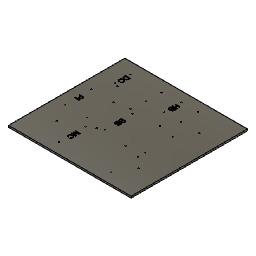
Bigger Board Tester v1 (Autodesk Fusion 360 design; units mm, degrees)
Autodesk Fusion 360 part; units mm, degrees
sketch "Sketch1" plane through (0, 0, 0) normal (0, 0, 1) x (1, 0, 0)
  circle A0 centre (-13.6792, 145.0658) radius 1.5
  circle A1 centre (165.3208, 145.0658) radius 1.5
  circle A2 centre (-13.6792, 12.1658) radius 1.5
  circle A3 centre (165.3208, 12.1658) radius 1.5
  circle A4 centre (43.3208, 42.5182) radius 1.5
  circle A5 centre (108.3208, 41.4658) radius 1.5
  circle A6 centre (43.3208, 116.7382) radius 1.5
  circle A7 centre (108.3208, 115.7658) radius 1.5
  line L0 (-58.5792, 206.1658) -> (210.2208, 206.1658)
  line L1 (210.2208, 206.1658) -> (210.2208, -48.9342)
  line L2 (210.2208, -48.9342) -> (-58.5792, -48.9342)
  line L3 (-58.5792, -48.9342) -> (-58.5792, 206.1658)
  dimension "d1" = 3
  dimension "d2" = 3
  dimension "d3" = 3
  dimension "d4" = 3
  dimension "d15" = 3
  dimension "d16" = 3
  dimension "d17" = 3
  dimension "d21" = 74.3
  dimension "d36" = 65
  dimension "d38" = 65
  dimension "d97" = 132.9
  dimension "d98" = 132.9
  dimension "d99" = 179
  dimension "d100" = 179
  dimension "d101" = 57
  dimension "d102" = 28.3275
  dimension "d106" = 61.1
  dimension "d107" = 61.1
  dimension "d108" = 44.9
  dimension "d109" = 44.9
  constraint horizontal L0
  constraint vertical L1
  constraint horizontal L2
  constraint vertical L3
  measures "d1" diameter of A0
  measures "d2" diameter of A1
  measures "d3" diameter of A2
  measures "d4" diameter of A3
  measures "d15" diameter of A5
  measures "d16" diameter of A6
  measures "d17" diameter of A7
  measures "d21" vertical distance of A5.centre A7.centre
  measures "d36" horizontal distance of A4.centre A5.centre
  measures "d38" horizontal distance of A6.centre A7.centre
  measures "d97" distance of A0.centre A2.centre
  measures "d98" distance of A1.centre A3.centre
  measures "d99" distance of A0.centre A1.centre
  measures "d100" distance of A2.centre A3.centre
  measures "d101" horizontal distance of A0.centre A6.centre
  measures "d102" vertical distance of A0.centre A6.centre
  measures "d106" distance of A2.centre L2
  measures "d107" distance of A0.centre L0
  measures "d108" distance of A0.centre L3
  measures "d109" distance of A1.centre L1
extrude "Extrude1" add sketch "Sketch1" along normal blind 3.5
sketch "Sketch2" plane through (0, 0, 3.5) normal (0, 0, 1) x (-1, 0, 0)
  circle A0 centre (-43.3208, -116.7382) radius 1.5
  circle A1 centre (-165.3208, -12.1658) radius 1.5
  circle A2 centre (-108.3208, -41.4658) radius 1.5
  circle A3 centre (13.6792, -12.1658) radius 1.5
  circle A4 centre (13.6792, -145.0658) radius 1.5
  circle A5 centre (-43.3208, -42.5182) radius 1.5
  circle A6 centre (-108.3208, -115.7658) radius 1.5
  circle A7 centre (-165.3208, -145.0658) radius 1.5
  line L0 (58.5792, 48.9342) -> (-210.2208, 48.9342)
  line L1 (-210.2208, 48.9342) -> (-210.2208, -206.1658)
  line L2 (-210.2208, -206.1658) -> (58.5792, -206.1658)
  line L3 (58.5792, -206.1658) -> (58.5792, 48.9342)
  line L4 (38.7881, -112.7975) -> (-15.0119, -112.7975)
  line L5 (-15.0119, -112.7975) -> (-15.0119, -49.6975)
  line L6 (-15.0119, -49.6975) -> (38.7881, -49.6975)
  line L7 (38.7881, -49.6975) -> (38.7881, -112.7975)
  circle A8 centre (36.2881, -110.2975) radius 1.25
  circle A9 centre (36.2881, -52.1975) radius 1.25
  circle A10 centre (-12.5119, -52.1975) radius 1.25
  circle A11 centre (-12.5119, -110.2975) radius 1.25
  line L8 (-145.573, 28.0042) -> (-25.813, 28.0042)
  line L9 (-145.573, -35.8758) -> (-145.573, 28.0042)
  circle A12 centre (-143.073, 25.5042) radius 1.25
  line L10 (-25.813, 28.0042) -> (-25.813, -35.8758)
  circle A13 centre (-143.073, -33.3758) radius 1.25
  circle A14 centre (-28.313, 25.5042) radius 1.25
  line L11 (-25.813, -35.8758) -> (-145.573, -35.8758)
  circle A15 centre (-28.313, -33.3758) radius 1.25
  line L12 (-125.9916, -186.7322) -> (-125.9916, -144.2322)
  line L13 (-84.6916, -186.7322) -> (-125.9916, -186.7322)
  circle A16 centre (-123.4916, -184.2322) radius 1.25
  line L14 (-125.9916, -144.2322) -> (-84.6916, -144.2322)
  circle A17 centre (-87.1916, -184.2322) radius 1.25
  circle A18 centre (-123.4916, -146.7322) radius 1.25
  line L15 (-84.6916, -144.2322) -> (-84.6916, -186.7322)
  circle A19 centre (-87.1916, -146.7322) radius 1.25
  line L16 (-145.6799, -111.5696) -> (-145.6799, -46.5696)
  line L17 (-52.6799, -111.5696) -> (-145.6799, -111.5696)
  circle A20 centre (-143.1799, -109.0696) radius 1.25
  line L18 (-145.6799, -46.5696) -> (-52.6799, -46.5696)
  circle A21 centre (-55.1799, -109.0696) radius 1.25
  circle A22 centre (-143.1799, -49.0696) radius 1.25
  line L19 (-52.6799, -46.5696) -> (-52.6799, -111.5696)
  circle A23 centre (-55.1799, -49.0696) radius 1.25
  line L20 (-49.2456, -183.6533) -> (-49.2456, -145.1533)
  line L21 (24.2544, -183.6533) -> (-49.2456, -183.6533)
  circle A24 centre (-46.7456, -181.1533) radius 1.25
  line L22 (-49.2456, -145.1533) -> (24.2544, -145.1533)
  circle A25 centre (21.7544, -181.1533) radius 1.25
  circle A26 centre (-46.7456, -147.6533) radius 1.25
  line L23 (24.2544, -145.1533) -> (24.2544, -183.6533)
  circle A27 centre (21.7544, -147.6533) radius 1.25
  dimension "d110" = 2.5
  dimension "d111" = 2.5
  dimension "d113" = 2.5
  dimension "d117" = 2.5
  dimension "d118" = 2.5
  dimension "d119" = 2.5
  dimension "d120" = 2.5
  dimension "d121" = 2.5
  dimension "d124" = 2.5
  dimension "d125" = 2.5
  dimension "d126" = 2.5
  dimension "d127" = 58.1
  dimension "d128" = 48.8
  dimension "d129" = 48.8
  dimension "d130" = 2.5
  dimension "d131" = 2.5
  dimension "d132" = 2.5
  dimension "d133" = 2.5
  dimension "d134" = 2.5
  dimension "d135" = 2.5
  dimension "d136" = 2.5
  dimension "d137" = 2.5
  dimension "d138" = 2.5
  dimension "d139" = 2.5
  dimension "d140" = 2.5
  dimension "d141" = 114.76
  dimension "d142" = 58.88
  dimension "d143" = 58.88
  dimension "d144" = 2.5
  dimension "d145" = 2.5
  dimension "d146" = 2.5
  dimension "d147" = 2.5
  dimension "d148" = 2.5
  dimension "d149" = 2.5
  dimension "d150" = 2.5
  dimension "d151" = 2.5
  dimension "d152" = 2.5
  dimension "d153" = 2.5
  dimension "d154" = 2.5
  dimension "d155" = 37.5
  dimension "d156" = 36.3
  dimension "d157" = 36.3
  dimension "d158" = 2.5
  dimension "d159" = 2.5
  dimension "d160" = 2.5
  dimension "d161" = 2.5
  dimension "d162" = 2.5
  dimension "d163" = 2.5
  dimension "d164" = 2.5
  dimension "d165" = 2.5
  dimension "d166" = 2.5
  dimension "d167" = 2.5
  dimension "d168" = 2.5
  dimension "d169" = 60
  dimension "d170" = 88
  dimension "d171" = 88
  dimension "d172" = 2.5
  dimension "d173" = 2.5
  dimension "d174" = 2.5
  dimension "d175" = 2.5
  dimension "d176" = 2.5
  dimension "d177" = 2.5
  dimension "d178" = 2.5
  dimension "d179" = 2.5
  dimension "d180" = 2.5
  dimension "d181" = 2.5
  dimension "d182" = 2.5
  dimension "d183" = 33.5
  dimension "d184" = 68.5
  dimension "d185" = 68.5
  dimension "d186" = 10
  dimension "d187" = 10
  dimension "d188" = 10
  dimension "d189" = 10
  dimension "d190" = 10
  dimension "d198" = 2.5
  dimension "d199" = 114.76
  text T0 "PI" font "Arial" height 10 align centre spacing 1 along the path L7 letters at x, y, angle (26.1414, -87.8471, 90) (26.1414, -78.5292, 90)
  text T1 "DC" font "Arial" height 10 align centre spacing 1 along the path L23 letters at x, y, angle (11.6077, -174.492, 90) (11.6077, -164.4033, 90)
  text T2 "HB" font "Arial" height 10 align centre spacing 1 along the path L15 letters at x, y, angle (-97.3383, -175.1855, 90) (-97.3383, -165.0968, 90)
  text T3 "BB" font "Arial" height 10 align centre spacing 1 along the path L19 letters at x, y, angle (-65.3266, -88.3874, 90) (-65.3266, -79.0696, 90)
  text T4 "MC" font "Arial" height 10 align centre spacing 1 along the path L10 letters at x, y, angle (-38.4596, -14.7987, 90) (-38.4596, -3.1616, 90)
  constraint horizontal L4
  constraint vertical L5
  constraint horizontal L6
  constraint vertical L7
  constraint horizontal L13
  constraint vertical L12
  constraint horizontal L14
  constraint vertical L15
  constraint horizontal L17
  constraint vertical L16
  constraint horizontal L18
  constraint vertical L19
  constraint horizontal L21
  constraint vertical L20
  constraint horizontal L22
  constraint vertical L23
  measures "d110" diameter of A8
  measures "d111" diameter of A9
  measures "d113" diameter of A10
  measures "d117" distance of L4 A8.centre
  measures "d118" distance of L7 A8.centre
  measures "d119" diameter of A11
  measures "d120" distance of L4 A11.centre
  measures "d121" distance of L5 A11.centre
  measures "d124" distance of L7 A9.centre
  measures "d125" distance of L6 A9.centre
  measures "d126" distance of L6 A10.centre
  measures "d127" distance of A8.centre A9.centre
  measures "d128" distance of A8.centre A11.centre
  measures "d129" distance of A9.centre A10.centre
  measures "d130" diameter of A13
  measures "d131" diameter of A15
  measures "d132" diameter of A14
  measures "d133" distance of A13.centre L9
  measures "d134" distance of A13.centre L11
  measures "d135" diameter of A12
  measures "d136" distance of A12.centre L9
  measures "d137" distance of A12.centre L8
  measures "d138" distance of A15.centre L11
  measures "d139" distance of A15.centre L10
  measures "d140" distance of A14.centre L10
  measures "d141" distance of A13.centre A15.centre
  measures "d142" distance of A12.centre A13.centre
  measures "d143" distance of A14.centre A15.centre
  measures "d144" diameter of A17
  measures "d145" diameter of A19
  measures "d146" diameter of A18
  measures "d147" distance of A17.centre L13
  measures "d148" distance of A17.centre L15
  measures "d149" diameter of A16
  measures "d150" distance of A16.centre L13
  measures "d151" distance of A16.centre L12
  measures "d152" distance of A19.centre L15
  measures "d153" distance of A19.centre L14
  measures "d154" distance of A18.centre L14
  measures "d155" distance of A17.centre A19.centre
  measures "d156" distance of A16.centre A17.centre
  measures "d157" distance of A18.centre A19.centre
  measures "d158" diameter of A21
  measures "d159" diameter of A23
  measures "d160" diameter of A22
  measures "d161" distance of A21.centre L17
  measures "d162" distance of A21.centre L19
  measures "d163" diameter of A20
  measures "d164" distance of A20.centre L17
  measures "d165" distance of A20.centre L16
  measures "d166" distance of A23.centre L19
  measures "d167" distance of A23.centre L18
  measures "d168" distance of A22.centre L18
  measures "d169" distance of A21.centre A23.centre
  measures "d170" distance of A20.centre A21.centre
  measures "d171" distance of A22.centre A23.centre
  measures "d172" diameter of A25
  measures "d173" diameter of A27
  measures "d174" diameter of A26
  measures "d175" distance of A25.centre L21
  measures "d176" distance of A25.centre L23
  measures "d177" diameter of A24
  measures "d178" distance of A24.centre L21
  measures "d179" distance of A24.centre L20
  measures "d180" distance of A27.centre L23
  measures "d181" distance of A27.centre L22
  measures "d182" distance of A26.centre L22
  measures "d183" distance of A25.centre A27.centre
  measures "d184" distance of A24.centre A25.centre
  measures "d185" distance of A26.centre A27.centre
  measures "d198" distance of A14.centre L8
  measures "d199" distance of A14.centre A12.centre
extrude "Extrude2" add sketch "Sketch2" along normal blind 0.5 text T0
extrude "Extrude3" add sketch "Sketch2" along normal blind 0.5 text T1
extrude "Extrude4" add sketch "Sketch2" along normal blind 0.5 text T2
extrude "Extrude5" add sketch "Sketch2" along normal blind 0.5 text T3
extrude "Extrude6" add sketch "Sketch2" along normal blind 0.5 text T4
extrude "Extrude7" cut sketch "Sketch2" against normal blind 3.5 contours A8 | A9 | A10 | A11 | A12 | A13 | A14 | A15 | A16 | A17 | A18 | A19 | A20 | A21 | A22 | A23 | A24 | A25 | A26 | A27
equation "d199 = d141"
